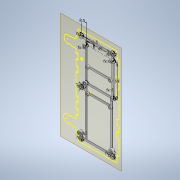
# Autodesk Inventor part: system_holder_plastic
Saved by Autodesk Inventor 2020 (Build 240168000, 168)
## iProperties
Created: 2020-01-14
Part Number: system_holder_plastic
Material: Generic
Document SubType Name: Modeling
Designer: erwin
Density: 1 g/cm^3
Appearance: Default
Author: erwin
Autodesk Inventor part; units mm, degrees
ref_plane "YZ Plane" through (0, 0, 0) normal (1, 0, 0) x (0, 1, 0)
ref_plane "XZ Plane" through (0, 0, 0) normal (0, 1, 0) x (-1, 0, 0)
ref_plane "XY Plane" through (0, 0, 0) normal (0, 0, 1) x (1, 0, 0)
ref_plane "Work Plane1" through (0, 0, 0) normal (0, 0, 1) x (1, 0, 0)
sketch "Sketch1" plane through (0, 0, 0) normal (0, 0, 1) x (1, 0, 0)
  circle A0 centre (-17, 43.4) radius 1.9
  circle A1 centre (-17, 79.8) radius 1.9
  circle A2 centre (39, -79.8) radius 1.9
  circle A3 centre (-17, -79.8) radius 1.9
  circle A4 centre (39, 79.8) radius 1.9
  circle A5 centre (-17, 0) radius 1.9
  circle A6 centre (39, 43.4) radius 1.9 construction
  arc A7 (-25.979899, 38.2) -> (-24, 40.179899) centre (-24.989949, 39.189949) ccw
  line L0 (-25.979899, 38.2) -> (-27.6, 38.2)
  line L1 (-27.6, 28.2) -> (-27.6, 38.2)
  line L2 (-27.6, 28.2) -> (-25.979899, 28.2)
  arc A8 (-24, 26.220101) -> (-25.979899, 28.2) centre (-24.989949, 27.210051) ccw
  line L3 (-24, 26.220101) -> (-24, 20.179899)
  arc A9 (-25.979899, 18.2) -> (-24, 20.179899) centre (-24.989949, 19.189949) ccw
  line L4 (-25.979899, 18.2) -> (-27.6, 18.2)
  line L5 (-27.6, -18.2) -> (-27.6, 18.2)
  line L6 (-27.6, -18.2) -> (-25.979899, -18.2)
  arc A10 (-24, -20.179899) -> (-25.979899, -18.2) centre (-24.989949, -19.189949) ccw
  line L7 (-24, -20.179899) -> (-24, -26.220101)
  arc A11 (-25.979899, -28.2) -> (-24, -26.220101) centre (-24.989949, -27.210051) ccw
  line L8 (-25.979899, -28.2) -> (-27.6, -28.2)
  line L9 (-27.6, -38.2) -> (-27.6, -28.2)
  line L10 (-27.6, -38.2) -> (-25.979899, -38.2)
  arc A12 (-24, -40.179899) -> (-25.979899, -38.2) centre (-24.989949, -39.189949) ccw
  line L11 (-24, -40.179899) -> (-24, -46.220101)
  arc A13 (-25.979899, -48.2) -> (-24, -46.220101) centre (-24.989949, -47.210051) ccw
  line L12 (-25.979899, -48.2) -> (-27.6, -48.2)
  line L13 (-27.6, -54.6) -> (-27.6, -48.2)
  line L14 (-36.995861, -54.6) -> (-27.6, -54.6)
  line L15 (-36.99445, -55.599999) -> (-36.995861, -54.6)
  line L16 (-40.99445, -55.599999) -> (-36.99445, -55.599999)
  line L17 (-40.995861, -54.6) -> (-40.99445, -55.599999)
  line L18 (-42.6, -54.6) -> (-40.995861, -54.6)
  arc A14 (-42.6, -54.6) -> (-42.6, -68.6) centre (-42.6, -61.6) ccw
  line L19 (-40.97611, -68.6) -> (-42.6, -68.6)
  line L20 (-40.973592, -67.600003) -> (-40.97611, -68.6)
  line L21 (-36.973592, -67.600003) -> (-40.973592, -67.600003)
  line L22 (-36.97611, -68.6) -> (-36.973592, -67.600003)
  line L23 (-27.6, -68.6) -> (-36.97611, -68.6)
  line L24 (-27.6, -75) -> (-27.6, -68.6)
  line L25 (-27.6, -75) -> (-25.979899, -75)
  arc A15 (-24, -76.979899) -> (-25.979899, -75) centre (-24.989949, -75.989949) ccw
  line L26 (-24, -76.979899) -> (-24, -86.8)
  line L27 (-24, -86.8) -> (46, -86.8)
  line L28 (46, -86.8) -> (46, -76.979899)
  arc A16 (47.979899, -75) -> (46, -76.979899) centre (46.989949, -75.989949) ccw
  line L29 (47.979899, -75) -> (49.6, -75)
  line L30 (49.6, -48.2) -> (49.6, -75)
  line L31 (49.6, -48.2) -> (47.979899, -48.2)
  arc A17 (46, -46.220101) -> (47.979899, -48.2) centre (46.989949, -47.210051) ccw
  line L32 (46, -46.220101) -> (46, -40.179899)
  arc A18 (47.979899, -38.2) -> (46, -40.179899) centre (46.989949, -39.189949) ccw
  line L33 (47.979899, -38.2) -> (49.6, -38.2)
  line L34 (49.6, -28.2) -> (49.6, -38.2)
  line L35 (49.6, -28.2) -> (47.979899, -28.2)
  arc A19 (46, -26.220101) -> (47.979899, -28.2) centre (46.989949, -27.210051) ccw
  line L36 (46, -26.220101) -> (46, -20.179899)
  arc A20 (47.979899, -18.2) -> (46, -20.179899) centre (46.989949, -19.189949) ccw
  line L37 (47.979899, -18.2) -> (49.6, -18.2)
  line L38 (49.6, 18.2) -> (49.6, -18.2)
  line L39 (49.6, 18.2) -> (47.979899, 18.2)
  arc A21 (46, 20.179899) -> (47.979899, 18.2) centre (46.989949, 19.189949) ccw
  line L40 (46, 20.179899) -> (46, 26.220101)
  arc A22 (47.979899, 28.2) -> (46, 26.220101) centre (46.989949, 27.210051) ccw
  line L41 (47.979899, 28.2) -> (49.6, 28.2)
  line L42 (49.6, 38.2) -> (49.6, 28.2)
  line L43 (49.6, 38.2) -> (47.979899, 38.2)
  arc A23 (46, 40.179899) -> (47.979899, 38.2) centre (46.989949, 39.189949) ccw
  line L44 (46, 40.179899) -> (46, 46.220101)
  arc A24 (47.979899, 48.2) -> (46, 46.220101) centre (46.989949, 47.210051) ccw
  line L45 (47.979899, 48.2) -> (49.6, 48.2)
  line L46 (49.6, 75) -> (49.6, 48.2)
  line L47 (49.6, 75) -> (47.979899, 75)
  arc A25 (46, 76.979899) -> (47.979899, 75) centre (46.989949, 75.989949) ccw
  line L48 (46, 76.979899) -> (46, 86.8)
  line L49 (46, 86.8) -> (-24, 86.8)
  line L50 (-24, 86.8) -> (-24, 76.979899)
  arc A26 (-25.979899, 75) -> (-24, 76.979899) centre (-24.989949, 75.989949) ccw
  line L51 (-25.979899, 75) -> (-27.6, 75)
  line L52 (-27.6, 68.6) -> (-27.6, 75)
  line L53 (-36.6, 68.6) -> (-27.6, 68.6)
  line L54 (-36.6, 67.6) -> (-36.6, 68.6)
  line L55 (-40.6, 67.6) -> (-36.6, 67.6)
  line L56 (-40.6, 68.6) -> (-40.6, 67.6)
  line L57 (-41.616274, 68.6) -> (-40.6, 68.6)
  arc A27 (-41.616274, 68.6) -> (-41.616274, 54.6) centre (-41.616274, 61.6) ccw
  line L58 (-40.6, 54.6) -> (-41.616274, 54.6)
  line L59 (-40.6, 55.6) -> (-40.6, 54.6)
  line L60 (-36.6, 55.6) -> (-40.6, 55.6)
  line L61 (-36.6, 54.6) -> (-36.6, 55.6)
  line L62 (-27.6, 54.6) -> (-36.6, 54.6)
  line L63 (-27.6, 48.2) -> (-27.6, 54.6)
  line L64 (-27.6, 48.2) -> (-25.979899, 48.2)
  arc A28 (-24, 46.220101) -> (-25.979899, 48.2) centre (-24.989949, 47.210051) ccw
  line L65 (-24, 46.220101) -> (-24, 40.179899)
  circle A29 centre (-17, 79.8) radius 1.7
  circle A30 centre (39, 79.8) radius 1.7
  circle A31 centre (-17, 0) radius 1.7
  circle A32 centre (-17, -79.8) radius 1.7
  circle A33 centre (39, -79.8) radius 1.7
  circle A34 centre (-17, 79.8) radius 3.7
  circle A35 centre (39, 79.8) radius 3.7
  circle A36 centre (-17, 0) radius 3.7
  circle A37 centre (-17, -79.8) radius 3.7
  circle A38 centre (39, -79.8) radius 3.7
  line L66 (-8.5, 11.3) -> (40.5, 11.3) construction
  line L67 (40.5, 11.3) -> (40.5, 69.3) construction
  line L68 (40.5, 69.3) -> (-8.5, 69.3) construction
  line L69 (-8.5, 69.3) -> (-8.5, 11.3) construction
  circle A39 centre (-8.5, 11.3) radius 3
  circle A40 centre (-8.5, 69.3) radius 3
  circle A41 centre (40.5, 11.3) radius 3
  circle A42 centre (40.5, 69.3) radius 3
  point P0 (0, 0)
  dimension "d0" = 0.2
  dimension "d1" = 0.2
  dimension "d2" = 0.2
  dimension "d3" = 0.2
  dimension "d4" = 0.2
  dimension "border" = 2
  dimension "d6" = 2
  dimension "d7" = 2
  dimension "d8" = 2
  dimension "d9" = 2
  dimension "d10" = 49
  dimension "d11" = 58
  dimension "d12" = 8.5
  dimension "d13" = 10.5
  dimension "pi_stand" = 6
  dimension "d15" = 6
  dimension "d16" = 6
  dimension "d17" = 6
  constraints: 14 centre point, 8 end point, 4 coincident, 2 parallel, 1 horizontal, 1 perpendicular
  measures "d0" radial gap between concentric circles of A1 A29
  measures "d1" radial gap between concentric circles of A4 A30
  measures "d2" radial gap between concentric circles of A31 A5
  measures "d3" radial gap between concentric circles of A32 A3
  measures "d4" radial gap between concentric circles of A33 A2
  measures "border" radial gap between concentric circles of A29 A34
  measures "d6" radial gap between concentric circles of A30 A35
  measures "d7" radial gap between concentric circles of A31 A36
  measures "d8" radial gap between concentric circles of A32 A37
  measures "d9" radial gap between concentric circles of A33 A38
  measures "d10" distance of L68.end L67.end
  measures "d11" distance of L67.end L66.end
  measures "d12" distance from line of A1.centre L69
  measures "d13" distance from line of A1.centre L68
  measures "pi_stand" diameter of A39
  measures "d15" diameter of A40
  measures "d16" diameter of A41
  measures "d17" diameter of A42
extrude "Extrusion1" add sketch "Sketch1" along normal blind 1 contours A1 | A2 | A3 | A4 | A5 | A34 | A35 | A36 | A37 | A38 | A39 | A40 | A41 | A42
sketch "Sketch2" plane through (0, 0, 0) normal (0, 0, 1) x (1, 0, 0)
  circle A0 centre (39, 79.8) radius 1.7
  circle A1 centre (39, 79.8) radius 3.7
  circle A2 centre (-17, 0) radius 1.7
  circle A3 centre (-17, 0) radius 3.7
  circle A4 centre (-17, -79.8) radius 1.7
  circle A5 centre (-17, -79.8) radius 3.7
  circle A6 centre (40.5, 69.3) radius 3
  circle A7 centre (-8.5, 69.3) radius 3
  circle A8 centre (40.5, 11.3) radius 3
  circle A9 centre (39, -79.8) radius 1.7
  circle A10 centre (39, -79.8) radius 3.7
  circle A11 centre (-8.5, 11.3) radius 3
  circle A12 centre (-17, 79.8) radius 1.7
  circle A13 centre (-17, 79.8) radius 3.7
  line L0 (38.327268, 69.3) -> (41.327268, 69.3)
  line L1 (41.327268, 69.3) -> (41.327268, 77.184282)
  line L2 (41.327268, 77.184282) -> (38.327268, 77.184282)
  line L3 (38.327268, 77.184282) -> (38.327268, 69.3)
  circle A14 centre (-17, 79.8) radius 3.7
  line L4 (36.697046, 80.444708) -> (-14.146476, 80.444708)
  line L5 (-14.146476, 80.444708) -> (-14.146476, 77.444708)
  line L6 (-14.146476, 77.444708) -> (36.697046, 77.444708)
  line L7 (36.697046, 77.444708) -> (36.697046, 80.444708)
  line L8 (-9.818631, 79.135677) -> (-6.818631, 79.135677)
  line L9 (-6.818631, 79.135677) -> (-6.818631, 10.753482)
  line L10 (-6.818631, 10.753482) -> (-9.818631, 10.753482)
  line L11 (-9.818631, 10.753482) -> (-9.818631, 79.135677)
  circle A15 centre (40.5, 69.3) radius 3
  line L12 (38.327268, 71.368632) -> (41.327268, 71.368632)
  line L13 (41.327268, 71.368632) -> (41.327268, 11.3)
  line L14 (41.327268, 11.3) -> (38.327268, 11.3)
  line L15 (38.327268, 11.3) -> (38.327268, 71.368632)
  line L16 (41.327268, 12.05766) -> (-9.818631, 12.05766)
  line L17 (-9.818631, 12.05766) -> (-9.818631, 9.05766)
  line L18 (-9.818631, 9.05766) -> (41.327268, 9.05766)
  line L19 (41.327268, 9.05766) -> (41.327268, 12.05766)
  line L20 (36.697046, -79.8) -> (-17, -79.8)
  line L21 (-17, -79.8) -> (-17, -76.8)
  line L22 (-17, -76.8) -> (36.697046, -76.8)
  line L23 (36.697046, -76.8) -> (36.697046, -79.8)
  line L24 (-6.818631, 9.873514) -> (-9.818631, 9.873514)
  line L25 (-9.818631, 9.873514) -> (-9.818631, -78.3)
  line L26 (-9.818631, -78.3) -> (-6.818631, -78.3)
  line L27 (-6.818631, -78.3) -> (-6.818631, 9.873514)
  circle A16 centre (-17, 0) radius 3.7
  line L28 (-14.146476, -2.355292) -> (-8.087264, -2.355292)
  line L29 (-8.087264, -2.355292) -> (-8.087264, 0.644708)
  line L30 (-8.087264, 0.644708) -> (-14.146476, 0.644708)
  line L31 (-14.146476, 0.644708) -> (-14.146476, -2.355292)
  line L32 (39, -78.1) -> (36, -78.1)
  line L33 (36, -78.1) -> (36, 11.6)
  line L34 (36, 11.6) -> (39, 11.6)
  line L35 (39, 11.6) -> (39, -78.1)
  point P0 (0, 0)
  point P1 (-6.818631, 77.444708)
  point P2 (-9.818631, 77.444708)
  point P3 (-9.818631, 0.644708)
  point P4 (-13.356602, 0.644708)
  point P5 (-9.818631, -2.355292)
  point P6 (-9.818631, -76.8)
  point P7 (-17, -78.1)
  point P8 (-15.3, -79.8)
  point P9 (-6.818631, -76.8)
  point P10 (-6.818631, 9.05766)
  point P11 (38.327268, 12.05766)
  point P12 (-6.818631, 12.05766)
  point P13 (39, 9.05766)
  point P14 (36, 9.05766)
  point P15 (36, -76.8)
  point P16 (36.697046, -78.1)
  dimension "d20" = 3
  dimension "d21" = 3
  dimension "d22" = 3
  dimension "d23" = 3
  dimension "d24" = 3
  dimension "d25" = 3
  dimension "d26" = 3
  dimension "d32" = 3
  constraints: 72 end point, 18 parallel, 9 horizontal, 9 perpendicular, 7 point on line, 1 vertical alignment, 7 other
  measures "d20" distance of L2.end L1.end
  measures "d21" distance of L5.end L4.end
  measures "d22" distance of L9.end L10.end
  measures "d23" distance of L17.end L16.end
  measures "d24" distance of L20.end L21.end
  measures "d25" distance of L26.end L25.end
  measures "d26" distance of L29.end L28.end
  measures "d32" distance of L33.end L34.end
move faces "Move1" translate (0, 0, 5) faces at (-8.842968, 10.731098, 1) (-7.722431, 69.723807, 1) (39.666003, 70.667161, 1) (41.414514, 10.595961, 1)
extrude "Extrusion2" add sketch "Sketch2" along normal blind 1 contours L4 L7 L6 A1 | A1 L6 L9 L8 L11 A13 L4 | L1 A6 L3 A1 | A1 L3 L2 L1 | A13 L5 L4 | L1 L12 A6 | L9 A7 L11 L6 | L6 L11 L8 L9 | L12 L1 L0 L3 | L9 A7 L11 | L15 L0 L13 A6 | A6 L13 A8 L15 | L9 A11 L11 A7 | A8 L13 L16 L15 | L9 L16 L11 A11 | L16 L15 L34 A8 | A8 L34 L33 L18 A11 L16 | L16 L13 L14 L35 L34 L15 | A11 L18 L27 L24 L17 L10 L9 L16 | L9 L10 L11 L16 | L34 L15 L14 L35 L18 A8 | A8 L18 L33 L34 | L34 L35 L14 L15 | L35 A10 L23 L22 L33 L18 A8 | A8 L18 L35 | L19 L18 L35 L14 | L25 L18 L27 A11 | A11 L27 L22 L25 L28 L29 L30 | L35 L32 L23 A10 | L17 L24 L27 L18 | L30 L29 L28 L25 | L25 L28 A3 L30 | L23 L32 L33 A10 | A10 L33 L22 L23 | L27 L26 L25 L22 | L22 L33 A10 L20 A5 L25 L26 L27 | A10 L33 L32 L23 L20 | L20 A4 L21 L22 A5 picked at (-13.992533, 78.682242) picked at (-16.032252, -77.289451)
sketch "Sketch3" plane through (40.5, 11.3, 6) normal (0, 0, 1) x (1, 0, 0)
  circle A0 centre (0, 0) radius 3 projected
  circle A1 centre (-49, 0) radius 3 projected
  circle A2 centre (-49, 58) radius 3 projected
  circle A3 centre (0, 58) radius 3 projected
  point P0 (-40.5, -11.3)
  constraints: 4 coincident
hole "Hole1" at (40.5, 11.3, 6) at (-8.5, 11.3, 6) at (-8.5, 69.3, 6) at (40.5, 69.3, 6) direction (0, 0, -1) diameter 2.5 end through all
sketch "Sketch4" plane through (0, 0, 0) normal (0, 0, 1) x (1, 0, 0)
  circle A0 centre (-4.25, -4.45) radius 2.744283
  circle A1 centre (-4.25, 37.55) radius 2.744283
  circle A2 centre (36.25, 37.55) radius 2.744283
  circle A3 centre (36.25, -4.45) radius 2.744283
  circle A4 centre (36.25, -4.45) radius 1.35
  circle A5 centre (36.25, 37.55) radius 1.35
  circle A6 centre (-4.25, 37.55) radius 1.35
  circle A7 centre (-4.25, -4.45) radius 1.35
  line L0 (36.25, 37.55) -> (-4.25, 37.55) construction
  line L1 (-4.25, 37.55) -> (-4.25, -4.45) construction
  line L2 (-4.25, -4.45) -> (36.25, -4.45) construction
  line L3 (36.25, -4.45) -> (36.25, 37.55) construction
  circle A8 centre (40.5, 11.3) radius 1.25 construction
  circle A9 centre (40.5, 11.3) radius 3 construction
  circle A10 centre (-8.5, 11.3) radius 1.25 construction
  point P0 (0, 0)
  dimension "d40" = 17
  dimension "d41" = 42
  dimension "d42" = 40.5
  dimension "d43" = 4.25
  dimension "d44" = 4.25
  constraints: 8 centre point, 8 end point, 5 coincident, 2 parallel, 1 horizontal, 1 perpendicular
  measures "d41" distance of L2.end L0.start
  measures "d42" distance between parallel lines of L1 L3
  measures "d43" distance from line of A9.centre L3
  measures "d44" distance from line of L1 A10.centre
extrude "Extrusion3" add sketch "Sketch4" along normal blind 4 contours A0 | A1 | A2 | A3 | A4 | A5 | A6 | A7
sketch "Sketch5" plane through (36.25, 37.55, 4) normal (0, 0, 1) x (1, 0, 0)
  circle A0 centre (0, 0) radius 2.744283 construction
  circle A1 centre (-40.5, 0) radius 2.744283 construction
  circle A2 centre (-40.5, -42) radius 2.744283 construction
  circle A3 centre (0, -42) radius 2.744283 construction
  point P0 (-36.25, -37.55)
  point P1 (-40.5, 0)
  point P2 (-40.5, -42)
  point P3 (0, -42)
  constraints: 4 coincident
hole "Hole2" at (36.25, 37.55, 4) at (-4.25, 37.55, 4) at (-4.25, -4.45, 4) at (36.25, -4.45, 4) direction (0, 0, -1) diameter 2.5 end through all
sketch "Sketch6" plane through (36.25, -4.45, 4) normal (0, 0, 1) x (1, 0, 0)
  circle A0 centre (0, 0) radius 1.25
  circle A1 centre (-40.5, 0) radius 1.25
  line L0 (0, 0) -> (-40.5, 0)
  line L1 (-20.25, 0) -> (-20.25, 27.327193) construction
  line L2 (2.75, 21.027577) -> (-43.25, 21.027577)
  line L3 (-43.25, 21.027577) -> (-43.25, 10.742489)
  line L4 (-43.25, 10.742489) -> (2.75, 10.742489)
  line L5 (2.75, 10.742489) -> (2.75, 21.027577)
  line L6 (2.75, 21.027577) -> (-43.25, 10.742489) construction
  line L7 (-43.25, 21.027577) -> (2.75, 10.742489) construction
  point P0 (-36.25, 4.45)
  point P1 (-20.25, 15.885033)
  dimension "d54" = 46
  constraints: 16 end point, 3 midpoint, 2 horizontal, 2 parallel, 1 perpendicular, 1 point on line, 1 vertical
  measures "d54" distance of L4.end L3.end
extrude "Extrusion4" cut sketch "Sketch6" along normal blind 4 contours L5 L4 L3 L2
sketch "Sketch7" plane through (0, 0, 0) normal (0, 0, -1) x (-1, 0, 0)
  circle A0 centre (4.25, -4.45) radius 2.744283
  line L0 (-35.031288, -5.000606) -> (3.012439, -5.000606)
  line L1 (3.012439, -5.000606) -> (3.012439, -2.000606)
  line L2 (3.012439, -2.000606) -> (-35.031288, -2.000606)
  line L3 (-35.031288, -2.000606) -> (-35.031288, -5.000606)
  line L4 (-34.473764, 35.876813) -> (3.25, 35.876813)
  line L5 (3.25, 35.876813) -> (3.25, 38.876813)
  line L6 (3.25, 38.876813) -> (-34.473764, 38.876813)
  line L7 (-34.473764, 38.876813) -> (-34.473764, 35.876813)
  point P0 (0, 0)
  dimension "d57" = 3
  dimension "d58" = 3
  constraints: 16 end point, 4 parallel, 2 horizontal, 2 perpendicular, 2 other
  measures "d57" distance of L1.end L0.end
  measures "d58" distance of L5.end L4.end
extrude "Extrusion5" add sketch "Sketch7" against normal blind 1 contours L1 L0 A0 | A0 L0 L3 L2 | L7 L6 L5 L4 picked at (2.845978, -3.108856)
sketch "Sketch8" plane through (0, 0, 0) normal (0, 0, -1) x (-1, 0, 0)
  line L0 (8.312822, 36.13708) -> (5.409124, 36.13708)
  line L1 (5.409124, 36.13708) -> (5.409124, 39.13708)
  line L2 (5.409124, 39.13708) -> (8.312822, 39.13708)
  line L3 (8.312822, 39.13708) -> (8.312822, 36.13708)
  line L4 (5.409124, -5.230445) -> (7.828556, -5.230445)
  line L5 (7.828556, -5.230445) -> (7.828556, -2.230445)
  line L6 (7.828556, -2.230445) -> (5.409124, -2.230445)
  line L7 (5.409124, -2.230445) -> (5.409124, -5.230445)
  point P0 (0, 0)
  dimension "d61" = 3
  dimension "d62" = 3
  constraints: 16 end point, 4 parallel, 2 horizontal, 2 perpendicular
  measures "d61" distance of L0.end L1.end
  measures "d62" distance of L5.end L4.end
extrude "Extrusion6" add sketch "Sketch8" against normal blind 1
sketch "Sketch9" plane through (0, 0, 0) normal (0, 0, 1) x (1, 0, 0)
  circle A0 centre (39, -79.8) radius 1.7 construction
  circle A1 centre (-17, -79.8) radius 1.7 construction
  line L0 (39, -79.8) -> (-17, -79.8) construction
  line L1 (-17, -79.8) -> (-17, -69.8) construction
  line L2 (-17, -69.8) -> (39, -69.8) construction
  line L3 (39, -69.8) -> (39, -79.8) construction
  circle A2 centre (39, -69.8) radius 3.4
  circle A3 centre (-17, -69.8) radius 3.4
  point P0 (0, 0)
  dimension "d65" = 10
  dimension "d66" = 6.8
  dimension "d67" = 6.8
  constraints: 8 end point, 2 centre point, 2 coincident, 2 parallel, 1 horizontal, 1 perpendicular
  measures "d65" distance of L0.end L1.end
  measures "d66" diameter of A2
  measures "d67" diameter of A3
extrude "Extrusion7" add sketch "Sketch9" along normal blind 4
sketch "Sketch10" plane through (0, 0, 0) normal (0, 0, -1) x (-1, 0, 0)
  line L0 (17.280838, -68.685421) -> (7.980048, -68.685421)
  line L1 (7.980048, -68.685421) -> (7.980048, -71.685421)
  line L2 (7.980048, -71.685421) -> (17.280838, -71.685421)
  line L3 (17.280838, -71.685421) -> (17.280838, -68.685421)
  line L4 (17.954808, -70.185421) -> (14.954808, -70.185421)
  line L5 (14.954808, -70.185421) -> (14.954808, -78.185421)
  line L6 (14.954808, -78.185421) -> (17.954808, -78.185421)
  line L7 (17.954808, -78.185421) -> (17.954808, -70.185421)
  point P0 (0, 0)
  point P1 (14.954808, -71.685421)
  point P2 (17.280838, -70.185421)
  dimension "d70" = 3
  dimension "d71" = 3
  dimension "d72" = 8
  constraints: 16 end point, 4 parallel, 2 horizontal, 2 perpendicular
  measures "d70" distance of L1.end L0.end
  measures "d71" distance of L6.end L5.end
  measures "d72" distance of L5.end L4.end
extrude "Extrusion8" add sketch "Sketch10" against normal blind 1
sketch "Sketch11" plane through (39, -69.8, 4) normal (0, 0, 1) x (1, 0, 0)
  circle A0 centre (0, 0) radius 3.4 projected
  circle A1 centre (-56, 0) radius 3.4 projected
  point P0 (-39, 69.8)
  constraints: 2 coincident
hole "Hole3" at (39, -69.8, 4) at (-17, -69.8, 4) direction (0, 0, -1) diameter 2.5 end through all
move faces "Move2" translate (0, 0, -1) faces at (-2.033431, -4.71914, 4) (-2.033431, 37.28086, 4) (38.466569, 37.28086, 4) (38.466569, -4.71914, 4) (-6.830869, 10.556855, 4) (38.187824, 10.95798, 4)
move faces "Move3" translate (0, 0, -2) faces at (-10.884571, 69.589539, 6) (38.115429, 69.589539, 6) (39.086371, 11.249776, 6) (-7.086371, 11.249776, 6)
chamfer "Chamfer1" distance 0.5 angle 45 10 edges at (-8.5, 70.55, 4) (40.5, 70.55, 4) (36.25, 38.8, 3) (-4.25, 38.8, 3) (-8.5, 12.55, 4) (-4.25, -3.2, 3) (36.25, -3.2, 3) (40.5, 12.55, 4) (39, -68.55, 4) (-17, -68.55, 4)
sketch "Sketch12" plane through (0, 0, 1) normal (0, 0, 1) x (1, 0, 0)
  point P0 (0, 0)
sketch "Sketch13" plane through (0, 0, 1) normal (0, 0, 1) x (1, 0, 0)
  circle A0 centre (39, -69.8) radius 1.25
  circle A1 centre (-17, -69.8) radius 1.25
  arc A2 (-14.834359, -76.8) -> (-14.954808, -76.716627) centre (-17, -79.8) ccw
  line L0 (-9.818631, -76.8) -> (-14.834359, -76.8)
  line L1 (-9.818631, -71.685421) -> (-9.818631, -76.8)
  line L2 (-9.818631, -71.685421) -> (-14.170656, -71.685421)
  arc A3 (-14.954808, -72.516099) -> (-14.170656, -71.685421) centre (-17, -69.8) ccw
  line L3 (-14.954808, -72.516099) -> (-14.954808, -76.716627)
  line L4 (-17.954808, -76.225319) -> (-17.954808, -73.06318)
  arc A4 (-13.78788, -68.685421) -> (-17.954808, -73.06318) centre (-17, -69.8) ccw
  line L5 (-13.78788, -68.685421) -> (-9.818631, -68.685421)
  line L6 (-9.818631, -2.355292) -> (-9.818631, -68.685421)
  line L7 (-14.146476, -2.355292) -> (-9.818631, -2.355292)
  arc A5 (-13.356602, 0.644708) -> (-14.146476, -2.355292) centre (-17, 0) ccw
  line L8 (-9.818631, 0.644708) -> (-13.356602, 0.644708)
  line L9 (-9.818631, 8.605336) -> (-9.818631, 0.644708)
  arc A6 (-9.818631, 13.994664) -> (-9.818631, 8.605336) centre (-8.5, 11.3) ccw
  line L10 (-9.818631, 66.605336) -> (-9.818631, 13.994664)
  arc A7 (-9.818631, 71.994664) -> (-9.818631, 66.605336) centre (-8.5, 69.3) ccw
  line L11 (-9.818631, 77.444708) -> (-9.818631, 71.994664)
  line L12 (-14.146476, 77.444708) -> (-9.818631, 77.444708)
  arc A8 (-13.356602, 80.444708) -> (-14.146476, 77.444708) centre (-17, 79.8) ccw
  line L13 (35.356602, 80.444708) -> (-13.356602, 80.444708)
  arc A9 (41.327268, 76.923575) -> (35.356602, 80.444708) centre (39, 79.8) ccw
  line L14 (41.327268, 72.183683) -> (41.327268, 76.923575)
  arc A10 (41.327268, 66.416317) -> (41.327268, 72.183683) centre (40.5, 69.3) ccw
  line L15 (41.327268, 14.183683) -> (41.327268, 66.416317)
  arc A11 (39, 8.701924) -> (41.327268, 14.183683) centre (40.5, 11.3) ccw
  line L16 (39, -66.4) -> (39, 8.701924)
  arc A12 (39, -73.2) -> (39, -66.4) centre (39, -69.8) ccw
  line L17 (39, -76.1) -> (39, -73.2)
  arc A13 (35.3, -79.8) -> (39, -76.1) centre (39, -79.8) ccw
  line L18 (-13.3, -79.8) -> (35.3, -79.8)
  arc A14 (-17.954808, -76.225319) -> (-13.3, -79.8) centre (-17, -79.8) ccw
  arc A15 (-17.532104, -78.185421) -> (-16.467896, -78.185421) centre (-17, -79.8) ccw
  line L19 (-16.467896, -78.185421) -> (-17.532104, -78.185421)
  line L20 (36, -7.182872) -> (36, -68.2)
  arc A16 (33.561521, -5.000606) -> (36, -7.182872) centre (36.25, -4.45) ccw
  line L21 (33.561521, -5.000606) -> (-1.561521, -5.000606)
  arc A17 (-6.818631, -5.416036) -> (-1.561521, -5.000606) centre (-4.25, -4.45) ccw
  line L22 (-6.818631, -76.8) -> (-6.818631, -5.416036)
  line L23 (36, -76.8) -> (-6.818631, -76.8)
  line L24 (36, -71.4) -> (36, -76.8)
  arc A18 (36, -68.2) -> (36, -71.4) centre (39, -69.8) ccw
  arc A19 (-1.847781, 38.876813) -> (-6.488809, 39.13708) centre (-4.25, 37.55) ccw
  line L25 (-1.847781, 38.876813) -> (33.847781, 38.876813)
  arc A20 (38.327268, 39.343333) -> (33.847781, 38.876813) centre (36.25, 37.55) ccw
  line L26 (38.327268, 67.231368) -> (38.327268, 39.343333)
  arc A21 (38.327268, 71.368632) -> (38.327268, 67.231368) centre (40.5, 69.3) ccw
  line L27 (38.327268, 76.161672) -> (38.327268, 71.368632)
  arc A22 (36.146476, 77.444708) -> (38.327268, 76.161672) centre (39, 79.8) ccw
  line L28 (-6.818631, 77.444708) -> (36.146476, 77.444708)
  line L29 (-6.818631, 71.784552) -> (-6.818631, 77.444708)
  arc A23 (-6.818631, 66.815448) -> (-6.818631, 71.784552) centre (-8.5, 69.3) ccw
  line L30 (-6.818631, 39.13708) -> (-6.818631, 66.815448)
  line L31 (-6.818631, 39.13708) -> (-6.488809, 39.13708)
  arc A24 (-3.012439, -2.000606) -> (-5.863897, -2.230445) centre (-4.25, -4.45) ccw
  line L32 (-3.012439, -2.000606) -> (35.012439, -2.000606)
  arc A25 (36, -1.717128) -> (35.012439, -2.000606) centre (36.25, -4.45) ccw
  line L33 (36, 9.05766) -> (36, -1.717128)
  line L34 (-6.507035, 9.05766) -> (36, 9.05766)
  arc A26 (-6.818631, 8.815448) -> (-6.507035, 9.05766) centre (-8.5, 11.3) ccw
  line L35 (-6.818631, -2.230445) -> (-6.818631, 8.815448)
  line L36 (-6.818631, -2.230445) -> (-5.863897, -2.230445)
  line L37 (-6.602604, 36.13708) -> (-6.818631, 36.13708)
  line L38 (-6.818631, 13.784552) -> (-6.818631, 36.13708)
  arc A27 (-5.597251, 12.05766) -> (-6.818631, 13.784552) centre (-8.5, 11.3) ccw
  line L39 (37.597251, 12.05766) -> (-5.597251, 12.05766)
  arc A28 (38.327268, 13.368632) -> (37.597251, 12.05766) centre (40.5, 11.3) ccw
  line L40 (38.327268, 35.756667) -> (38.327268, 13.368632)
  arc A29 (34.074791, 35.876813) -> (38.327268, 35.756667) centre (36.25, 37.55) ccw
  line L41 (34.074791, 35.876813) -> (-2.074791, 35.876813)
  arc A30 (-6.602604, 36.13708) -> (-2.074791, 35.876813) centre (-4.25, 37.55) ccw
  arc A31 (-5.409124, 37.082098) -> (-3.25, 36.8) centre (-4.25, 37.55) ccw
  arc A32 (-5.409124, -4.917902) -> (-3.012439, -4.625905) centre (-4.25, -4.45) ccw
  circle A33 centre (36.25, 37.55) radius 1.25
  arc A34 (35.031288, -4.727922) -> (35.031288, -4.172078) centre (36.25, -4.45) ccw
  circle A35 centre (-8.5, 69.3) radius 1.25
  circle A36 centre (40.5, 11.3) radius 1.25
  circle A37 centre (-8.5, 11.3) radius 1.25
  circle A38 centre (40.5, 69.3) radius 1.25
  circle A39 centre (-17, 0) radius 1.7
  circle A40 centre (39, -79.8) radius 1.7
  circle A41 centre (-17, 79.8) radius 1.7
  circle A42 centre (39, 79.8) radius 1.7
  circle A43 centre (39, 79.8) radius 3.7
  circle A44 centre (-17, 79.8) radius 3.7
  circle A45 centre (-17, 0) radius 3.7
  circle A46 centre (39, -79.8) radius 3.7
  arc A47 (-17.954808, -76.225319) -> (-13.3, -79.8) centre (-17, -79.8) ccw
  circle A48 centre (-17, -79.8) radius 3.7
  line L42 (-3.012439, -4.625905) -> (-3.012439, -4.274095)
  arc A49 (-3.012439, -4.274095) -> (-5.409124, -3.982098) centre (-4.25, -4.45) ccw
  line L43 (-5.409124, -3.982098) -> (-5.409124, -4.917902)
  line L44 (35.031288, -4.172078) -> (35.031288, -4.727922)
  line L45 (-3.25, 36.8) -> (-3.25, 38.3)
  arc A50 (-3.25, 38.3) -> (-5.409124, 38.017902) centre (-4.25, 37.55) ccw
  line L46 (-5.409124, 38.017902) -> (-5.409124, 37.082098)
  point P0 (0, 0)
extrude "Extrusion9" add sketch "Sketch13" along normal blind 1 contours A48 A14 A2 | A46 A13 | A5 A45 | A43 A22 A9 | A44 A8
delete faces "Delete Face1" heal yes whole lump no faces at (-17.177368, -78.185421, 0.666667) (-16.822632, -78.185421, 1.666667)
equation "\"d1\" = d0"
equation "\"d2\" = d0"
equation "\"d3\" = d0"
equation "\"d4\" = d0"
equation "\"d6\" = border"
equation "\"d7\" = border"
equation "\"d8\" = border"
equation "\"d9\" = border"
equation "\"d15\" = pi_stand"
equation "\"d16\" = pi_stand"
equation "\"d17\" = pi_stand"
equation "\"d43\" = d44"
equation "\"d67\" = d66"
body "Solid1"
